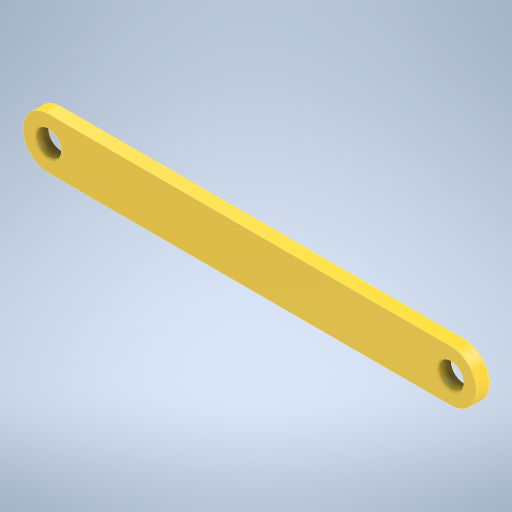
# Autodesk Inventor part: 2-HUDSON-8-32-TDR HAND PUMP LINK
Saved by Autodesk Inventor 2024.2 (Build 282272000, 272)
## iProperties
Created: 2024-11-02
Part Number: 2-HUDSON-8-32-TDR HAND PUMP LINK
Material: Genérico
Document SubType Name: Modeling
Designer: brene
Density: 1 g/cm^3
Appearance: Brillante - Oro
Author: brene
Autodesk Inventor part; units mm, degrees
ref_plane "YZ Plane" through (0, 0, 0) normal (1, 0, 0) x (0, 1, 0)
ref_plane "XZ Plane" through (0, 0, 0) normal (0, 1, 0) x (-1, 0, 0)
ref_plane "XY Plane" through (0, 0, 0) normal (0, 0, 1) x (1, 0, 0)
sketch "Boceto1" plane through (0, 0, 0) normal (0, 0, 1) x (1, 0, 0)
  line L0 (-31.5, 8) -> (31.5, 8)
  line L1 (31.5, 8) -> (31.5, 0)
  line L2 (31.5, 0) -> (-31.5, 0)
  line L3 (-31.5, 0) -> (-31.5, 8)
  arc A0 (-31.5, 8) -> (-31.5, 0) centre (-31.5, 4) ccw
  arc A1 (31.5, 0) -> (31.5, 8) centre (31.5, 4) ccw
  circle A2 centre (-31.5, 4) radius 2
  circle A3 centre (31.5, 4) radius 2
  point P0 (0, 0)
  point P1 (0, 0)
  dimension "d0" = 8
  dimension "d3" = 63
  dimension "d4" = 4
  dimension "d5" = 4
  constraints: 8 end point, 4 centre point, 4 point on circle, 3 coincident, 3 midpoint, 2 parallel, 1 horizontal, 1 perpendicular
  measures "d0" distance of L2.end L0.start
  measures "d3" distance of A1.centre A0.centre
  measures "d4" diameter of A3
  measures "d5" diameter of A2
extrude "Extrusión1" add sketch "Boceto1" along normal blind 2 contours L0 L1 A3 L2 L3 A2 | L3 A2 A0 | A1 L1 A3
equation "\"d5\" = d4"
